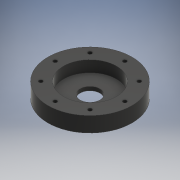
# Autodesk Inventor part: CS02
Saved by Autodesk Inventor 2017 (Build 210142000, 142)
## iProperties
Created: 2019-11-06
Part Number: CS02
Material: ABS Plastic
Document SubType Name: Modeling
Designer: Dell
Density: 1.06 g/cm^3
Appearance: Smooth - Black
Author: Dell
Autodesk Inventor part; units mm, degrees
ref_plane "YZ Plane" through (0, 0, 0) normal (1, 0, 0) x (0, 1, 0)
ref_plane "XZ Plane" through (0, 0, 0) normal (0, 1, 0) x (-1, 0, 0)
ref_plane "XY Plane" through (0, 0, 0) normal (0, 0, 1) x (1, 0, 0)
sketch "Sketch1" plane through (0, 0, 0) normal (0, 0, 1) x (1, 0, 0)
  circle A0 centre (0, 0) radius 13
  circle A1 centre (0, 0) radius 55.5
  dimension "d0" = 26
  dimension "d1" = 111
  constraints: 2 centre point, 2 coincident
  measures "d0" diameter of A0
  measures "d1" diameter of A1
extrude "Extrusion1" add sketch "Sketch1" along normal blind 5
sketch "Sketch2" plane through (0, 0, 5) normal (0, 0, 1) x (1, 0, 0)
  circle A0 centre (0, 0) radius 35
  circle A1 centre (0, 0) radius 55.5 projected
  dimension "d4" = 70
  constraints: 1 centre point, 1 coincident
  measures "d4" diameter of A0
extrude "Extrusion2" add sketch "Sketch2" along normal blind 15
sketch "Sketch3" plane through (0, 0, 0) normal (0, 0, -1) x (-1, 0, 0)
  circle A0 centre (0, 0) radius 39.5
  circle A1 centre (0, 0) radius 53
  dimension "d7" = 79
  dimension "d8" = 106
  constraints: 2 centre point, 2 coincident
  measures "d7" diameter of A0
  measures "d8" diameter of A1
extrude "Extrusion3" cut sketch "Sketch3" against normal blind 3
chamfer "Chamfer1" distance 2 angle 15 1 edges at (39.5, 0, 3) measured on face at (39.5, 0, 2.5)
chamfer "Chamfer2" distance 2 angle 15 1 edges at (53, 0, 3) measured on face at (53, 0, 2.5)
sketch "Sketch5" plane through (0, 0, 20) normal (0, 0, 1) x (1, 0, 0)
  circle A0 centre (-46, 0) radius 2.5
  circle A1 centre (-32.5269, -32.5269) radius 2.5
  circle A2 centre (0, -46) radius 2.5
  circle A3 centre (32.5269, -32.5269) radius 2.5
  circle A4 centre (46, 0) radius 2.5
  circle A5 centre (32.5269, 32.5269) radius 2.5
  circle A6 centre (0, 46) radius 2.5
  circle A7 centre (-32.5269, 32.5269) radius 2.5
  point P0 (0, 0)
  dimension "d17" = 5
  dimension "d18" = 46
  dimension "d21" = 360
  constraints: 8 centre point, 1 horizontal alignment, 17 other
  measures "d17" diameter of A0
  measures "d18" distance of A0.centre point (0, 0)
extrude "Extrusion4" cut sketch "Sketch5" against normal through all
sketch "Sketch6" plane through (0, 0, 3) normal (0, 0, -1) x (-1, 0, 0)
  circle A0 centre (-46, 0) radius 2.5 projected
  line L0 (-46, -5.1962) -> (-50.5, -2.5981)
  line L1 (-50.5, -2.5981) -> (-50.5, 2.5981)
  line L2 (-50.5, 2.5981) -> (-46, 5.1962)
  line L3 (-46, 5.1962) -> (-41.5, 2.5981)
  line L4 (-41.5, 2.5981) -> (-41.5, -2.5981)
  line L5 (-41.5, -2.5981) -> (-46, -5.1962)
  line L6 (-28.8527, -36.2011) -> (-33.8718, -37.546)
  line L7 (-33.8718, -37.546) -> (-37.546, -33.8718)
  line L8 (-37.546, -33.8718) -> (-36.2011, -28.8527)
  line L9 (-36.2011, -28.8527) -> (-31.182, -27.5078)
  line L10 (-31.182, -27.5078) -> (-27.5078, -31.182)
  line L11 (-27.5078, -31.182) -> (-28.8527, -36.2011)
  line L12 (5.1962, -46) -> (2.5981, -50.5)
  line L13 (2.5981, -50.5) -> (-2.5981, -50.5)
  line L14 (-2.5981, -50.5) -> (-5.1962, -46)
  line L15 (-5.1962, -46) -> (-2.5981, -41.5)
  line L16 (-2.5981, -41.5) -> (2.5981, -41.5)
  line L17 (2.5981, -41.5) -> (5.1962, -46)
  line L18 (36.2011, -28.8527) -> (37.546, -33.8718)
  line L19 (37.546, -33.8718) -> (33.8718, -37.546)
  line L20 (33.8718, -37.546) -> (28.8527, -36.2011)
  line L21 (28.8527, -36.2011) -> (27.5078, -31.182)
  line L22 (27.5078, -31.182) -> (31.182, -27.5078)
  line L23 (31.182, -27.5078) -> (36.2011, -28.8527)
  line L24 (46, 5.1962) -> (50.5, 2.5981)
  line L25 (50.5, 2.5981) -> (50.5, -2.5981)
  line L26 (50.5, -2.5981) -> (46, -5.1962)
  line L27 (46, -5.1962) -> (41.5, -2.5981)
  line L28 (41.5, -2.5981) -> (41.5, 2.5981)
  line L29 (41.5, 2.5981) -> (46, 5.1962)
  line L30 (28.8527, 36.2011) -> (33.8718, 37.546)
  line L31 (33.8718, 37.546) -> (37.546, 33.8718)
  line L32 (37.546, 33.8718) -> (36.2011, 28.8527)
  line L33 (36.2011, 28.8527) -> (31.182, 27.5078)
  line L34 (31.182, 27.5078) -> (27.5078, 31.182)
  line L35 (27.5078, 31.182) -> (28.8527, 36.2011)
  line L36 (-5.1962, 46) -> (-2.5981, 50.5)
  line L37 (-2.5981, 50.5) -> (2.5981, 50.5)
  line L38 (2.5981, 50.5) -> (5.1962, 46)
  line L39 (5.1962, 46) -> (2.5981, 41.5)
  line L40 (2.5981, 41.5) -> (-2.5981, 41.5)
  line L41 (-2.5981, 41.5) -> (-5.1962, 46)
  line L42 (-36.2011, 28.8527) -> (-37.546, 33.8718)
  line L43 (-37.546, 33.8718) -> (-33.8718, 37.546)
  line L44 (-33.8718, 37.546) -> (-28.8527, 36.2011)
  line L45 (-28.8527, 36.2011) -> (-27.5078, 31.182)
  line L46 (-27.5078, 31.182) -> (-31.182, 27.5078)
  line L47 (-31.182, 27.5078) -> (-36.2011, 28.8527)
  point P0 (0, 0)
  point P1 (-32.5269, -32.5269)
  point P2 (0, -46)
  point P3 (32.5269, -32.5269)
  point P4 (46, 0)
  point P5 (32.5269, 32.5269)
  point P6 (0, 46)
  point P7 (-32.5269, 32.5269)
  dimension "d25" = 9
  dimension "d28" = 360
  constraints: 96 end point, 1 coincident, 1 vertical, 118 other
  measures "d25" distance between parallel lines of L4 L1
extrude "Extrusion5" cut sketch "Sketch6" against normal blind 4.5 contours A0 | L0 L1 L2 L3 L4 L5 | L6 L7 L8 L9 L10 L11 | L12 L13 L14 L15 L16 L17 | L18 L19 L20 L21 L22 L23 | L24 L25 L26 L27 L28 L29 | L30 L31 L32 L33 L34 L35 | L36 L37 L38 L39 L40 L41 | L42 L43 L44 L45 L46 L47
body "Solid1"
